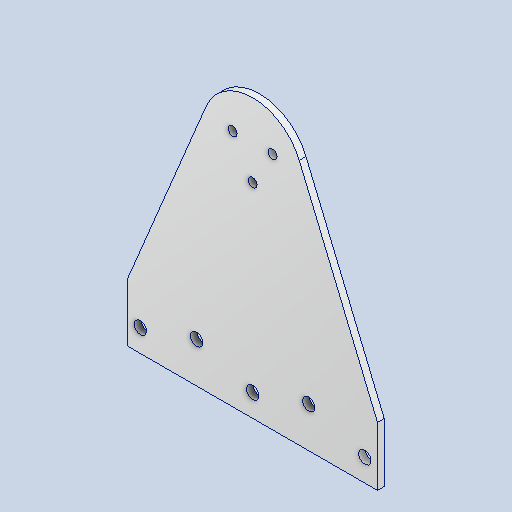
# Autodesk Inventor part: BLACHA_2_Przegub
Saved by Autodesk Inventor 2023 (Build 270158000, 158)
## iProperties
Created: 2023-02-13
Part Number: BLACHA_2_Przegub
Material: Aluminium 6061
Document SubType Name: Modeling
Designer: Kamil
Density: 2.7 g/cm^3
Appearance: Aluminium — płaski
Author: Kamil
Autodesk Inventor part; units mm, degrees
ref_plane "YZ Plane" through (0, 0, 0) normal (1, 0, 0) x (0, 1, 0)
ref_plane "XZ Plane" through (0, 0, 0) normal (0, 1, 0) x (-1, 0, 0)
ref_plane "XY Plane" through (0, 0, 0) normal (0, 0, 1) x (1, 0, 0)
sketch "Szkic1" plane through (0, 0, 0) normal (0, 0, 1) x (1, 0, 0)
  circle A0 centre (55.6246, 7) radius 2.75 projected
  circle A1 centre (30.6246, 15) radius 2.75 projected
  circle A2 centre (80.6246, 15) radius 2.75 projected
  circle A3 centre (5.6246, 7) radius 2.75 projected
  circle A4 centre (105.6246, 7) radius 2.75 projected
  line L0 (111.2491, 0) -> (0, 0) projected
  line L1 (111.2491, 0) -> (111.2491, 23.25) projected
  line L2 (0, 23.25) -> (111.2491, 23.25) projected
  line L3 (0, 0) -> (0, 23.25) projected
  line L4 (55.6245, 23.25) -> (55.6245, 98.25)
  circle A5 centre (55.6245, 98.25) radius 22.5
  line L5 (111.2491, 23.25) -> (24.4674, 231.5289)
  line L6 (0, 23.25) -> (68.7685, 188.2966)
  point P0 (76.3938, 106.9037)
  point P1 (34.8553, 106.9037)
  dimension "d0" = 75
  dimension "d1" = 98.25
  dimension "d2" = 45
  constraints: 6 end point, 2 coincident, 2 tangent, 1 centre point, 1 midpoint, 1 vertical
  measures "d0" distance of L4.start L4.end
  measures "d1" vertical distance of L0.end L4.end
  measures "d2" diameter of A5
extrude "Wyciągnięcie proste1" add sketch "Szkic1" along normal blind 3 contours L0 L3 L2 L1 | L2 L4 A5 L5 | L6 A5 L4 L2 | A5
sketch "Szkic2" plane through (0, 0, 3) normal (0, 0, 1) x (1, 0, 0)
  line L0 (34.8553, 106.9037) -> (0, 23.25) projected
  line L1 (0, 23.25) -> (0, 0) projected
  line L2 (0, 0) -> (111.2491, 0) projected
  line L3 (111.2491, 0) -> (111.2491, 23.25) projected
  line L4 (111.2491, 23.25) -> (76.3938, 106.9037) projected
  arc A0 (76.3938, 106.9037) -> (34.8553, 106.9037) centre (55.6245, 98.25) ccw projected
  circle A1 centre (105.6246, 7) radius 2.75 projected
  circle A2 centre (5.6246, 7) radius 2.75 projected
  circle A3 centre (80.6246, 15) radius 2.75 projected
  circle A4 centre (30.6246, 15) radius 2.75 projected
  circle A5 centre (55.6246, 7) radius 2.75 projected
  line L5 (55.6245, 98.25) -> (55.6245, 88)
  circle A6 centre (55.6245, 88) radius 2
  circle A7 centre (64.5013, 103.375) radius 2
  circle A8 centre (46.7478, 103.375) radius 2
  dimension "d5" = 10.25
  dimension "d6" = 4
  dimension "d9" = 360
  constraints: 3 centre point, 2 end point, 1 coincident, 1 vertical, 7 other
  measures "d5" distance of L5.start L5.end
  measures "d6" diameter of A6
extrude "Wyciągnięcie proste2" cut sketch "Szkic2" against normal through all contours A6 | A7 | A8
move faces "Przesuń1" translate (0, -3, 0) faces at (37.083, 0, 1)
